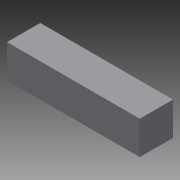
# Autodesk Inventor part: Tubebase
Saved by Autodesk Inventor 2015 (Build 190159000, 159)
## iProperties
Created: 2016-05-27
Part Number: Tubebase
Material: Generic
Document SubType Name: Modeling
Designer: Toby
Density: 1 g/cm^3
Appearance: Default
Author: Toby
Autodesk Inventor part; units mm, degrees
ref_plane "YZ Plane" through (0, 0, 0) normal (1, 0, 0) x (0, 1, 0)
ref_plane "XZ Plane" through (0, 0, 0) normal (0, 1, 0) x (-1, 0, 0)
ref_plane "XY Plane" through (0, 0, 0) normal (0, 0, 1) x (1, 0, 0)
sketch "Sketch1" plane through (0, 0, 0) normal (0, 0, 1) x (1, 0, 0)
  line L0 (-53.4454, -1.4286) -> (-13.4454, -1.4286)
  line L1 (-13.4454, -1.4286) -> (-13.4454, -11.4286)
  line L2 (-13.4454, -11.4286) -> (-53.4454, -11.4286)
  line L3 (-53.4454, -11.4286) -> (-53.4454, -1.4286)
  circle A0 centre (-47.9454, -6.4286) radius 2.6
  circle A1 centre (-18.9454, -6.4286) radius 2.6
  point P0 (0, 0)
  dimension "d0" = 10
  dimension "d1" = 5.2
  dimension "d2" = 5.2
  dimension "d3" = 5
  dimension "d4" = 5
  dimension "d5" = 40
  dimension "d6" = 5.5
  dimension "d7" = 34.5
  constraints: 8 end point, 2 centre point, 2 parallel, 1 horizontal, 1 perpendicular
  measures "d0" distance of L2.end L0.start
  measures "d1" diameter of A0
  measures "d2" diameter of A1
  measures "d3" distance from line of L2 A0.centre
  measures "d4" distance from line of L2 A1.centre
  measures "d5" distance of L0.start L0.end
  measures "d6" distance from line of L3 A0.centre
  measures "d7" distance from line of L3 A1.centre
extrude "Extrusion1" add sketch "Sketch1" along normal blind 7
sketch "Sketch2" plane through (0, 0, 7) normal (0, 0, 1) x (1, 0, 0)
  line L0 (-53.4454, -1.4286) -> (-13.4454, -1.4286)
  line L1 (-13.4454, -1.4286) -> (-13.4454, -11.4286)
  line L2 (-13.4454, -11.4286) -> (-53.4454, -11.4286)
  line L3 (-53.4454, -11.4286) -> (-53.4454, -1.4286)
  point P0 (0, 0)
  constraints: 8 end point, 2 parallel, 1 horizontal, 1 perpendicular
extrude "Extrusion2" add sketch "Sketch2" along normal blind 3
body "Solid1"
